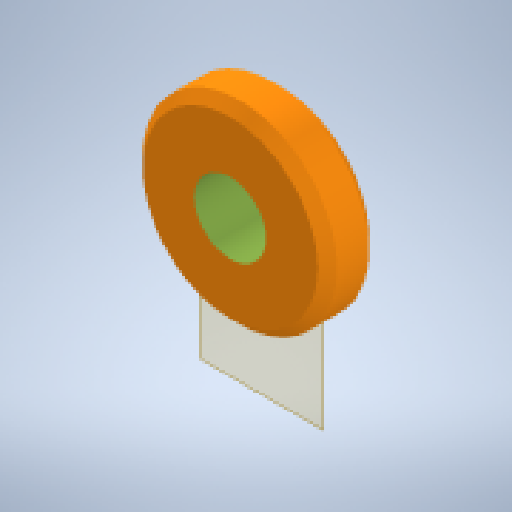
# Autodesk Inventor part: Wheel
Saved by Autodesk Inventor 2023 (Build 270158000, 158)
## iProperties
Created: 2023-11-24
Part Number: Wheel
Material: Generic
Document SubType Name: Modeling
Designer: danie
Density: 1 g/cm^3
Appearance: Olive Green
Author: danie
Autodesk Inventor part; units mm, degrees
ref_plane "YZ Plane" through (0, 0, 0) normal (1, 0, 0) x (0, 1, 0)
ref_plane "XZ Plane" through (0, 0, 0) normal (0, 1, 0) x (-1, 0, 0)
ref_plane "XY Plane" through (0, 0, 0) normal (0, 0, 1) x (1, 0, 0)
ref_plane "Work Plane1" through (-52.4749, 258.6532, -6.397) normal (0, 0, 1) x (0, -1, 0)
sketch "Sketch1" plane through (-52.4749, 258.6532, -6.397) normal (0, 0, 1) x (0, -1, 0)
  line L0 (0.0003, 0.0039) -> (-20.2411, 10.8651) projected
  arc A0 (-20.2411, 10.8651) -> (-35.6461, -2.9695) centre (-25.4455, 1.1661) ccw projected
  line L1 (-35.6461, -2.9695) -> (42.4229, -195.5278) projected
  line L2 (42.4229, -195.5278) -> (42.4229, -219.8278) projected
  line L3 (42.4229, -219.8278) -> (81.4481, -219.8278) projected
  line L4 (81.4481, -219.8278) -> (168.2058, -219.8263) projected
  line L5 (168.2058, -219.8263) -> (207.231, -219.8261) projected
  line L6 (207.231, -219.8261) -> (207.2309, -195.5273) projected
  ellipse E0 centre (186.2274, -195.5271) end of major axis (212.7883, -195.527) minor radius 0.0003 (207.231, -195.5268) -> (207.2309, -195.5273) ccw projected
  line L7 (207.231, -195.5268) -> (285.3, -2.9593) projected
  arc A1 (285.3, -2.9593) -> (269.9065, 10.8669) centre (275.106, 1.1734) ccw projected
  line L8 (269.9065, 10.8669) -> (249.6555, 0.0046) projected
  arc A2 (246.3474, -0.8266) -> (249.6555, 0.0046) centre (246.3474, 6.172) ccw projected
  line L9 (246.3474, -0.8266) -> (234.7987, -0.8277) projected
  arc A3 (234.7987, -0.8277) -> (224.1037, -11.8268) centre (235.1053, -11.8251) ccw projected
  line L10 (224.1037, -11.8268) -> (224.1037, -23.8268) projected
  line L11 (224.1037, -23.8268) -> (25.5516, -23.8268) projected
  line L12 (25.5516, -23.8268) -> (25.5516, -11.8268) projected
  arc A4 (25.5516, -11.8268) -> (14.3466, -0.8277) centre (14.5506, -11.8268) ccw projected
  line L13 (14.3466, -0.8277) -> (3.3091, -0.8277) projected
  arc A5 (0.0003, 0.0039) -> (3.3091, -0.8277) centre (3.3091, 6.1703) ccw projected
  circle A6 centre (275.1036, 1.1723) radius 4.5971 projected
  circle A7 centre (235.1053, -11.8251) radius 4.1019 projected
  circle A8 centre (14.5506, -11.8268) radius 4.101 projected
  circle A9 centre (61.9506, -207.5286) radius 4.1026 projected
  circle A10 centre (187.7028, -207.5216) radius 4.1055 projected
  circle A11 centre (-25.4489, 1.1708) radius 4.0986 projected
  circle A12 centre (-25.4489, 1.1708) radius 30
  point P0 (258.6534, 52.4739)
  dimension "d0" = 60
  constraints: 1 centre point, 1 coincident, 1 other
  measures "d0" diameter of A12
extrude "Extrusion1" add sketch "Sketch1" along normal blind 16 contours A5 L13 A12 L1 A0 L0 | L0 A0 L1 A12 L13 A5 | A11
chamfer "Chamfer1" distance 3 angle 45 2 edges at (-51.3043, 314.1021, -6.3967) (-51.3043, 314.102, 9.6033)
sketch "Sketch2" plane through (-51.3042, 284.102, 9.6032) normal (0, 0, 1) x (1, 0, 0)
  circle A0 centre (0, 0) radius 27 projected
  circle A1 centre (-0.0044, 0.002) radius 4.0977 projected
  circle A2 centre (-0.0044, 0.002) radius 11
  point P0 (51.3042, -284.102)
  dimension "d8" = 22
  constraints: 2 coincident, 1 centre point
  measures "d8" diameter of A2
extrude "Extrusion2" cut sketch "Sketch2" against normal through all contours A1 | A2
body "Solid1"
